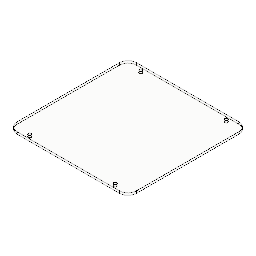
tock_thread_base_lid (Autodesk Fusion 360 design; units mm, degrees)
Autodesk Fusion 360 part; units mm, degrees
sketch "Sketch1" plane through (0, 0, 0) normal (0, 0, 1) x (1, 0, 0)
  line L0 (0, 0) -> (177.8, 0)
  line L1 (177.8, 0) -> (177.8, 177.8)
  line L2 (177.8, 177.8) -> (0, 177.8)
  line L3 (0, 177.8) -> (0, 0)
  dimension "d2" = 177.8
  dimension "d3" = 177.8
  constraint horizontal L0
  constraint vertical L1
  constraint horizontal L2
  constraint vertical L3
  constraint coincident L0.start L3.end
  measures "d2" distance of L0.start L0.end
  measures "d3" distance of L0.start L2.end
extrude "Extrude1" add sketch "Sketch1" along normal blind 3.175
fillet "Fillet1" radius 12.7 4 edges at (177.8, 0, 1.5875) (0, 0, 1.5875) (177.8, 177.8, 1.5875) (0, 177.8, 1.5875)
sketch "Sketch2" plane through (0, 0, 3.175) normal (0, 0, 1) x (-1, 0, 0)
  arc A0 (-12.7, -177.8) -> (0, -165.1) centre (-12.7, -165.1) ccw
  line L0 (0, -165.1) -> (0, -12.7)
  arc A1 (0, -12.7) -> (-12.7, 0) centre (-12.7, -12.7) ccw
  line L1 (-12.7, 0) -> (-165.1, 0)
  arc A2 (-165.1, 0) -> (-177.8, -12.7) centre (-165.1, -12.7) ccw
  line L2 (-177.8, -12.7) -> (-177.8, -165.1)
  arc A3 (-177.8, -165.1) -> (-165.1, -177.8) centre (-165.1, -165.1) ccw
  line L3 (-165.1, -177.8) -> (-12.7, -177.8)
  line L4 (-25.4, -171.45) -> (-152.4, -171.45) construction
  line L5 (-152.4, -171.45) -> (-152.4, -6.35) construction
  line L6 (-152.4, -6.35) -> (-25.4, -6.35) construction
  line L7 (-25.4, -6.35) -> (-25.4, -171.45) construction
  line L8 (-152.4, -100.0288) -> (-177.8, -100.0288) construction
  line L9 (-25.4, -101.0393) -> (0, -101.0393) construction
  line L10 (-70.6928, -171.45) -> (-70.6928, -177.8) construction
  line L11 (-68.6718, -6.35) -> (-68.6718, 0) construction
  circle A4 centre (-152.4, -6.35) radius 2.05
  dimension "d8" = 25.4
  dimension "d9" = 6.35
  dimension "d10" = 4.1
  constraint horizontal L4
  constraint vertical L5
  constraint horizontal L6
  constraint vertical L7
  constraint coincident L5 L8.start
  constraint coincident L2 L8.end
  constraint perpendicular L2 L8
  constraint coincident L7 L9.start
  constraint coincident L0 L9.end
  constraint perpendicular L0 L9
  constraint equal L8 L9
  constraint coincident L4 L10.start
  constraint coincident L3 L10.end
  constraint perpendicular L3 L10
  constraint coincident L6 L11.start
  constraint coincident L1 L11.end
  constraint perpendicular L1 L11
  constraint equal L10 L11
  constraint coincident L5.end L6.start
  measures "d8" distance of L2 L5
  measures "d9" distance of L1 L6
  measures "d10" diameter of A4
extrude "Extrude2" cut sketch "Sketch2" against normal through all contours A4
pattern_linear "R-Pattern1" count 2 spacing 127 along (-1, 0, 0) count 2 spacing 165.1 along (0, 1, 0) of "Extrude2"
equation "side = 7 in"
equation "d2 = side"
equation "d3 = side"
equation "d4 = ( 1 / 8 ) * 1 in"
